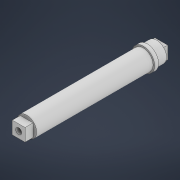
# Autodesk Inventor part: Verbindung_Rocker_Body
Saved by Autodesk Inventor 2021 (Build 250183000, 183)
## iProperties
Created: 2021-01-29
Part Number: Verbindung_Rocker_Body
Material: Generisch
Document SubType Name: Modeling
Designer: Ctroi
Density: 1 g/cm^3
Appearance: Vorgabe
Author: Ctroi
Autodesk Inventor part; units mm, degrees
ref_plane "YZ Plane" through (0, 0, 0) normal (1, 0, 0) x (0, 1, 0)
ref_plane "XZ Plane" through (0, 0, 0) normal (0, 1, 0) x (-1, 0, 0)
ref_plane "XY Plane" through (0, 0, 0) normal (0, 0, 1) x (1, 0, 0)
sketch "Skizze1" plane through (0, 0, 0) normal (0, 0, 1) x (1, 0, 0)
  line L0 (-4.75, 4.75) -> (4.75, 4.75)
  line L1 (4.75, 4.75) -> (4.75, -4.75)
  line L2 (4.75, -4.75) -> (-4.75, -4.75)
  line L3 (-4.75, -4.75) -> (-4.75, 4.75)
  line L4 (-4.75, 4.75) -> (4.75, -4.75) construction
  line L5 (4.75, 4.75) -> (-4.75, -4.75) construction
  point P0 (0, 0)
  dimension "d0" = 9.5
  dimension "d1" = 9.5
  constraints: 12 end point, 2 midpoint, 2 parallel, 1 horizontal, 1 perpendicular
  measures "d0" distance of L1.end L2.end
  measures "d1" distance of L0.end L1.end
extrude "Extrusion1" add sketch "Skizze1" along normal blind 3.5
sketch "Skizze2" plane through (0, 0, 3.5) normal (0, 0, 1) x (1, 0, 0)
  circle A0 centre (0, 0) radius 7.4
  dimension "d4" = 14.8
  constraints: 1 centre point, 1 coincident
  measures "d4" diameter of A0
extrude "Extrusion2" add sketch "Skizze2" along normal blind 7
sketch "Skizze7" plane through (0, 0, 10.5) normal (0, 0, 1) x (1, 0, 0)
  circle A0 centre (0, 0) radius 8.5
  dimension "d20" = 17
  constraints: 1 centre point, 1 coincident
  measures "d20" diameter of A0
extrude "Extrusion7" add sketch "Skizze7" along normal blind 3
sketch "Skizze8" plane through (0, 0, 13.5) normal (0, 0, 1) x (1, 0, 0)
  circle A0 centre (0, 0) radius 7.4
  dimension "d23" = 14.8
  constraints: 1 centre point, 1 coincident
  measures "d23" diameter of A0
extrude "Extrusion8" add sketch "Skizze8" along normal blind 87
sketch "Skizze9" plane through (0, 0, 100.5) normal (0, 0, 1) x (1, 0, 0)
  line L0 (4.75, 4.75) -> (-4.75, 4.75)
  line L1 (-4.75, 4.75) -> (-4.75, -4.75)
  line L2 (-4.75, -4.75) -> (4.75, -4.75)
  line L3 (4.75, -4.75) -> (4.75, 4.75)
  line L4 (4.75, 4.75) -> (-4.75, -4.75) construction
  line L5 (-4.75, 4.75) -> (4.75, -4.75) construction
  point P0 (0, 0)
  dimension "d26" = 9.5
  dimension "d27" = 9.5
  constraints: 12 end point, 2 midpoint, 2 parallel, 1 horizontal, 1 perpendicular
  measures "d26" distance of L2.end L1.end
  measures "d27" distance of L1.end L0.end
extrude "Extrusion9" add sketch "Skizze9" along normal blind 6
sketch "Skizze10" plane through (0, 0, 106.5) normal (0, 0, 1) x (1, 0, 0)
  circle A0 centre (0, 0) radius 2.25
  dimension "d30" = 4.5
  constraints: 1 centre point, 1 coincident
  measures "d30" diameter of A0
extrude "Extrusion10" cut sketch "Skizze10" against normal blind 5
sketch "Skizze11" plane through (0, 0, 0) normal (0, 0, -1) x (-1, 0, 0)
  circle A0 centre (0, 0) radius 2.25
  dimension "d33" = 4.5
  constraints: 1 centre point, 1 coincident
  measures "d33" diameter of A0
extrude "Extrusion11" cut sketch "Skizze11" against normal blind 5
